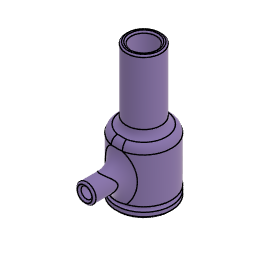
noiseMakerSimpleV2 (Autodesk Fusion 360 design; units mm, degrees)
Autodesk Fusion 360 part; units mm, degrees
note: some values were not read from the file. Chosen so that the rebuilt part matches the saved one: which face or edge a step refers to; which pieces of a blend or face edit are solid.
sketch "Sketch1" plane through (0, 0, 0) normal (0, 0, 1) x (1, 0, 0)
  circle A0 centre (0, 0) radius 17.5
  circle A1 centre (0, 0) radius 14
  circle A2 centre (0, 0) radius 11
  circle A3 centre (0, 0) radius 8
  dimension "d2" = 35
  dimension "d3" = 28
  dimension "d4" = 22
  dimension "d5" = 16
  constraint coincident A0.centre A1.centre
  constraint concentric A0 A1
  constraint concentric A1 A2
  constraint concentric A0 A3
  measures "d2" diameter of A0
  measures "d3" diameter of A1
  measures "d4" diameter of A2
  measures "d5" diameter of A3
extrude "Extrude7" add sketch "Sketch1" along normal blind 40 contours A0 makes body 1
extrude "Extrude8" add sketch "Sketch1" along normal blind 85 separate body contours A2 makes body 2
sketch "Sketch5" plane through (0, 0, 40) normal (0, 0, 1) x (-1, 0, 0)
  circle A0 centre (0, 0) radius 14
  circle A1 centre (0, 0) radius 17.5
  circle A2 centre (0, 0) radius 17.5
  circle A3 centre (0, 0) radius 11
  dimension "d60" = 35
  dimension "d61" = 22
  constraint concentric A0 A2
  constraint concentric A2 A3
  measures "d60" diameter of A2
  measures "d61" diameter of A3
extrude "Extrude9" add sketch "Sketch5" against normal blind 3 contours A0 | A1 A2 bodies 1 2
sketch "Sketch6" plane through (0, 0, 0) normal (1, 0, 0) x (0, 1, 0)
  circle A0 centre (17.4, 5) radius 1.5
  line L0 (17.5, 0) -> (-17.5, 0)
  dimension "d38" = 3
  dimension "d39" = 5
  dimension "d40" = 17.4
  measures "d38" diameter of A0
  measures "d39" distance of A0.centre L0
  measures "d40" horizontal distance of A0.centre origin
revolve "Revolve2" cut sketch "Sketch6" angle 360 about axis through (0, 0, 1.75) along (0, 0, 1) bodies 1
fillet "Fillet4" radius 1 1 edges at (-16.3157, -6.3283, 0) on bodies 1
ref_plane "WorkPlane1" through (0, -37.5, 0) normal (0, 1, 0) x (0, 0, 1)
sketch "Sketch7" plane through (0, -37.5, 0) normal (0, 1, 0) x (1, 0, 0)
  circle A0 centre (0, -20) radius 6
  circle A1 centre (0, -20) radius 3.5
  dimension "d45" = 12
  dimension "d46" = 20
  dimension "d47" = 7
  constraint concentric A0 A1
  measures "d45" diameter of A0
  measures "d46" distance of origin A0.centre
  measures "d47" diameter of A1
extrude "Extrude10" add sketch "Sketch7" along normal blind 23 contours A0 | A1 bodies 1
extrude "Extrude11" cut sketch "Sketch7" along normal blind 26 contours A1 bodies 1
fillet "Fillet5" radius 10 1 edges at (-6, -16.4393, 19.9909) on bodies 1
fillet "Fillet6" radius 1.2 2 edges at (-5.594, -37.5, 22.1697) (-3.2631, -37.5, 21.2657) on bodies 1
fillet "Fillet7" radius 5 2 edges at (-16.3157, -6.3283, 40) (-10.2556, -3.9778, 40) on bodies 1
fillet "Fillet8" radius 1 2 edges at (-7.4586, 2.8929, 85) (-10.2556, -3.9778, 85) on bodies 1 2
equation "ExternalDiam = 35 mm"
equation "d2 = ExternalDiam"
equation "d3 = ExternalDiam - 7 mm"
equation "d4 = ExternalDiam - 7 mm - 6 mm"
equation "d5 = ExternalDiam - 7 mm - 6 mm - 6 mm"
equation "OverallLength = 85 mm"
equation "d34 = OverallLength"
equation "d40 = ( ExternalDiam / 2 ) - 0.1 mm"
equation "d44 = -ExternalDiam / 2 - 20 mm"
equation "d60 = ExternalDiam"
equation "d61 = ExternalDiam - 13 mm"
